Autodesk Fusion 360 part; units mm, degrees
(part 2 of 4)
  arc A532 (19.4796, 24.4743) -> (19.5304, 24.4743) centre (19.505, 24.4743) ccw
  arc A533 (21.1153, 25.5016) -> (20.7851, 25.1714) centre (21.1153, 25.1714) ccw
  arc A534 (22.3677, 26.8884) -> (22.4113, 26.9145) centre (22.3895, 26.9015) ccw
  arc A535 (22.0907, 25.1714) -> (22.0399, 25.1714) centre (22.0653, 25.1714) ccw
  arc A536 (23.3454, 24.2062) -> (23.3454, 24.1554) centre (23.3454, 24.1808) ccw
  arc A537 (19.7985, 24.94) -> (19.7985, 24.8892) centre (19.7985, 24.9146) ccw
  arc A538 (19.505, 24.4743) -> (19.7985, 24.1808) centre (19.7985, 24.4743) ccw
  arc A539 (20.2387, 24.1554) -> (20.2387, 24.2062) centre (20.2387, 24.1808) ccw
  arc A540 (21.5189, 24.1554) -> (21.5189, 24.2062) centre (21.5189, 24.1808) ccw
  arc A541 (20.7851, 24.2062) -> (20.7851, 24.1554) centre (20.7851, 24.1808) ccw
  line L151 (22.3895, 26.9014) -> (21.9492, 27.6352)
  arc A542 (19.4796, 24.6211) -> (19.5304, 24.6211) centre (19.505, 24.6211) ccw
  arc A543 (21.5189, 25.2081) -> (21.1153, 25.5016) centre (21.1153, 25.0774) ccw
  arc A544 (19.7985, 24.9146) -> (19.505, 24.6211) centre (19.7985, 24.6211) ccw
  arc A545 (21.0582, 26.3144) -> (21.3517, 26.6079) centre (21.0582, 26.6079) ccw
  line L152 (19.7985, 24.9146) -> (20.2387, 24.9146)
  arc A546 (20.2641, 25.5016) -> (20.2133, 25.5016) centre (20.2387, 25.5016) ccw
  arc A547 (22.1578, 24.8962) -> (22.1929, 24.933) centre (22.1754, 24.9146) ccw
  arc A548 (23.4748, 24.931) -> (23.4361, 24.8981) centre (23.4554, 24.9145) ccw
  arc A549 (22.3955, 25.527) -> (22.3955, 25.4762) centre (22.3955, 25.5016) ccw
  line L153 (20.2387, 24.1808) -> (19.7985, 24.1808)
  line L154 (20.2387, 24.9146) -> (20.2387, 25.5016)
  arc A550 (22.3955, 25.5016) -> (22.0653, 25.1714) centre (22.3955, 25.1714) ccw
  line L155 (22.1753, 24.9146) -> (22.799, 24.1808)
  arc A551 (23.7377, 27.6352) -> (23.6869, 27.6352) centre (23.7123, 27.6352) ccw
  line L156 (23.4555, 24.9146) -> (24.0792, 24.1808)
  arc A552 (23.438, 24.8962) -> (23.473, 24.933) centre (23.4555, 24.9146) ccw
  arc A553 (24.0598, 24.1643) -> (24.0986, 24.1973) centre (24.0792, 24.1808) ccw
  line L157 (20.7647, 26.3144) -> (21.0582, 26.3144)
  arc A554 (21.9238, 26.3144) -> (21.9746, 26.3144) centre (21.9492, 26.3144) ccw
  line L158 (24.0792, 27.6352) -> (23.3454, 27.6352)
  line L159 (21.3517, 26.6079) -> (21.3517, 27.3417)
  arc A555 (20.7597, 25.1714) -> (20.8105, 25.1714) centre (20.7851, 25.1714) ccw
  arc A556 (27.0866, 42.545) -> (27.1818, 42.1322) centre (28.0285, 42.5448) ccw
  arc A557 (27.1749, 42.8823) -> (27.1253, 42.8427) centre (27.1501, 42.8625) ccw
  arc A558 (26.0673, 42.9438) -> (26.0103, 42.9717) centre (26.0388, 42.9578) ccw
  arc A559 (20.2387, 24.8892) -> (20.2387, 24.94) centre (20.2387, 24.9146) ccw
  line L160 (27.6581, 42.2275) -> (27.1501, 42.8625)
  arc A560 (26.5786, 42.545) -> (26.4833, 42.9578) centre (25.6366, 42.5449) ccw
  arc A561 (25.4419, 42.7355) -> (25.3784, 42.7355) centre (25.4102, 42.7355) ccw
  arc A562 (22.799, 25.2081) -> (22.3955, 25.5016) centre (22.3955, 25.0775) ccw
  arc A563 (26.4548, 42.1462) -> (26.5118, 42.1183) centre (26.4833, 42.1322) ccw
  arc A564 (22.799, 24.1554) -> (22.799, 24.2062) centre (22.799, 24.1808) ccw
  arc A565 (20.2133, 24.9146) -> (20.2641, 24.9146) centre (20.2387, 24.9146) ccw
  line L161 (20.2387, 25.5016) -> (19.505, 25.5016)
  arc A566 (26.4533, 42.9475) -> (26.5133, 42.968) centre (26.4833, 42.9577) ccw
  arc A567 (27.1183, 42.545) -> (27.0548, 42.545) centre (27.0866, 42.545) ccw
  arc A568 (27.2103, 42.9438) -> (27.1533, 42.9717) centre (27.1818, 42.9578) ccw
  line L162 (28.5471, 43.1165) -> (28.5471, 41.9735)
  line L163 (28.8646, 42.8625) -> (28.5471, 43.1165)
  arc A569 (25.9118, 42.545) -> (25.9753, 42.545) centre (25.9436, 42.545) ccw
  arc A570 (27.4041, 42.0053) -> (27.4041, 41.9417) centre (27.4041, 41.9735) ccw
  arc A571 (19.7985, 24.2062) -> (19.7985, 24.1554) centre (19.7985, 24.1808) ccw
  arc A572 (26.6103, 42.545) -> (26.5468, 42.545) centre (26.5785, 42.545) ccw
  arc A573 (27.7533, 42.545) -> (27.6898, 42.545) centre (27.7216, 42.545) ccw
  arc A574 (28.5669, 43.1413) -> (28.5272, 43.0917) centre (28.547, 43.1165) ccw
  arc A575 (27.4041, 43.1165) -> (27.1818, 42.9578) centre (27.404, 42.8816) ccw
  arc A576 (27.6898, 42.545) -> (27.7533, 42.545) centre (27.7216, 42.545) ccw
  arc A577 (27.6263, 42.1322) -> (27.7216, 42.545) centre (26.7796, 42.5451) ccw
  arc A578 (27.4041, 43.1483) -> (27.4041, 43.0847) centre (27.4041, 43.1165) ccw
  arc A579 (28.8447, 42.8377) -> (28.8844, 42.8873) centre (28.8646, 42.8625) ccw
  arc A580 (26.2611, 43.1165) -> (26.0388, 42.9578) centre (26.261, 42.8816) ccw
  arc A581 (27.0548, 42.545) -> (27.1183, 42.545) centre (27.0866, 42.545) ccw
  arc A582 (27.5978, 42.1462) -> (27.6548, 42.1183) centre (27.6263, 42.1322) ccw
  arc A583 (24.9339, 42.545) -> (24.8704, 42.545) centre (24.9022, 42.545) ccw
  arc A584 (21.4947, 25.2003) -> (21.5431, 25.2159) centre (21.5189, 25.2081) ccw
  arc A585 (20.7851, 25.1714) -> (20.8952, 24.9146) centre (21.1397, 25.1714) ccw
  arc A586 (27.1818, 42.9578) -> (27.0866, 42.545) centre (28.0285, 42.5452) ccw
  arc A587 (27.1518, 42.968) -> (27.2118, 42.9475) centre (27.1818, 42.9577) ccw
  arc A588 (27.4041, 41.9417) -> (27.4041, 42.0053) centre (27.4041, 41.9735) ccw
  arc A589 (27.5963, 42.9475) -> (27.6563, 42.968) centre (27.6263, 42.9577) ccw
  arc A590 (28.2296, 42.0053) -> (28.2296, 41.9417) centre (28.2296, 41.9735) ccw
  arc A591 (26.0388, 42.9578) -> (25.9436, 42.545) centre (26.8855, 42.5452) ccw
  line L164 (19.505, 24.4743) -> (19.505, 24.6211)
  arc A592 (26.4833, 42.1322) -> (26.5786, 42.545) centre (25.6366, 42.5451) ccw
  arc A593 (27.6263, 42.9578) -> (27.4041, 43.1165) centre (27.4041, 42.8816) ccw
  arc A594 (26.2611, 43.0847) -> (26.2611, 43.1483) centre (26.2611, 43.1165) ccw
  line L165 (24.13, 43.1165) -> (24.0665, 43.1165)
  arc A595 (27.6563, 42.122) -> (27.5963, 42.1425) centre (27.6263, 42.1322) ccw
  arc A596 (27.2118, 42.1425) -> (27.1518, 42.122) centre (27.1818, 42.1322) ccw
  arc A597 (28.5153, 41.9735) -> (28.5788, 41.9735) centre (28.5471, 41.9735) ccw
  arc A598 (27.1818, 42.1322) -> (27.4041, 41.9735) centre (27.404, 42.2084) ccw
  arc A599 (27.7216, 42.545) -> (27.6263, 42.9578) centre (26.7796, 42.5449) ccw
  arc A600 (27.4041, 41.9735) -> (27.6263, 42.1322) centre (27.4041, 42.2084) ccw
  arc A601 (26.4833, 42.9578) -> (26.2611, 43.1165) centre (26.2611, 42.8816) ccw
  arc A602 (27.6333, 42.2077) -> (27.6829, 42.2473) centre (27.6581, 42.2275) ccw
  arc A603 (26.2611, 43.1483) -> (26.2611, 43.0847) centre (26.2611, 43.1165) ccw
  arc A604 (26.0088, 42.968) -> (26.0688, 42.9475) centre (26.0388, 42.9577) ccw
  arc A605 (26.5468, 42.545) -> (26.6103, 42.545) centre (26.5785, 42.545) ccw
  arc A606 (26.5118, 42.9717) -> (26.4548, 42.9438) centre (26.4833, 42.9578) ccw
  line L166 (20.8952, 24.9146) -> (21.5189, 24.1808)
  arc A607 (27.1533, 42.1183) -> (27.2103, 42.1462) centre (27.1818, 42.1322) ccw
  arc A608 (27.4041, 43.0847) -> (27.4041, 43.1483) centre (27.4041, 43.1165) ccw
  arc A609 (28.5788, 43.1165) -> (28.5153, 43.1165) centre (28.5471, 43.1165) ccw
  arc A610 (28.8646, 41.9417) -> (28.8646, 42.0053) centre (28.8646, 41.9735) ccw
  line L167 (28.8646, 41.9735) -> (28.2296, 41.9735)
  arc A611 (27.6548, 42.9717) -> (27.5978, 42.9438) centre (27.6263, 42.9578) ccw
  arc A612 (27.1699, 47.8403) -> (27.1302, 47.7907) centre (27.1501, 47.8155) ccw
  arc A613 (24.0665, 47.625) -> (23.876, 47.8155) centre (23.876, 47.625) ccw
  arc A614 (25.9753, 42.545) -> (25.9118, 42.545) centre (25.9436, 42.545) ccw
  line L168 (27.1501, 47.8155) -> (27.1501, 46.6725)
  line L169 (26.5151, 42.2275) -> (26.0071, 42.8625)
  arc A615 (24.8704, 41.9735) -> (24.9339, 41.9735) centre (24.9022, 41.9735) ccw
  arc A616 (25.1879, 47.4345) -> (25.1244, 47.4345) centre (25.1562, 47.4345) ccw
  arc A617 (26.2293, 46.8313) -> (26.3246, 47.244) centre (25.3829, 47.2441) ccw
  arc A618 (25.7213, 47.244) -> (25.6578, 47.244) centre (25.6896, 47.244) ccw
  arc A619 (23.876, 47.7837) -> (23.876, 47.8473) centre (23.876, 47.8155) ccw
  arc A620 (26.0071, 46.6407) -> (26.0071, 46.7043) centre (26.0071, 46.6725) ccw
  arc A621 (25.7563, 46.8173) -> (25.8133, 46.8452) centre (25.7848, 46.8313) ccw
  arc A622 (24.0983, 47.625) -> (24.0348, 47.625) centre (24.0666, 47.625) ccw
  arc A623 (25.0927, 42.7037) -> (25.0927, 42.7673) centre (25.0927, 42.7355) ccw
  arc A624 (24.0348, 47.625) -> (24.0983, 47.625) centre (24.0666, 47.625) ccw
  arc A625 (23.8125, 47.8473) -> (23.8125, 47.7837) centre (23.8125, 47.8155) ccw
  arc A626 (24.4475, 42.7037) -> (24.4475, 42.7673) centre (24.4475, 42.7355) ccw
  arc A627 (23.876, 47.8473) -> (23.876, 47.7837) centre (23.876, 47.8155) ccw
  line L170 (27.4676, 47.5615) -> (27.1501, 47.8155)
  arc A628 (24.13, 43.0847) -> (24.13, 43.1483) centre (24.13, 43.1165) ccw
  line L171 (25.4102, 42.7355) -> (25.0927, 42.7355)
  line L172 (24.3205, 41.9735) -> (24.3205, 42.926)
  arc A629 (25.3784, 41.9735) -> (25.4419, 41.9735) centre (25.4102, 41.9735) ccw
  arc A630 (24.3523, 42.926) -> (24.2888, 42.926) centre (24.3206, 42.926) ccw
  arc A631 (26.4903, 42.2077) -> (26.5399, 42.2473) centre (26.5151, 42.2275) ccw
  line L173 (24.9022, 42.545) -> (24.9022, 41.9735)
  line L174 (24.4475, 42.7355) -> (24.0665, 42.7355)
  arc A632 (24.0665, 42.7673) -> (24.0665, 42.7037) centre (24.0665, 42.7355) ccw
  arc A633 (26.0388, 42.1322) -> (26.2611, 41.9735) centre (26.261, 42.2084) ccw
  line L175 (25.4102, 41.9735) -> (25.4102, 42.7355)
  arc A634 (24.8704, 42.545) -> (24.9339, 42.545) centre (24.9022, 42.545) ccw
  arc A635 (26.2611, 41.9735) -> (26.4833, 42.1322) centre (26.2611, 42.2084) ccw
  arc A636 (25.0927, 42.7673) -> (25.0927, 42.7037) centre (25.0927, 42.7355) ccw
  arc A637 (25.7779, 47.5813) -> (25.7283, 47.5417) centre (25.7531, 47.5615) ccw
  arc A638 (24.6482, 46.7043) -> (24.6482, 46.6407) centre (24.6482, 46.6725) ccw
  arc A639 (25.6896, 47.244) -> (25.7848, 46.8313) centre (26.6313, 47.2439) ccw
  arc A640 (25.8133, 47.6428) -> (25.7563, 47.6707) centre (25.7848, 47.6567) ccw
  arc A641 (24.2888, 41.9735) -> (24.3523, 41.9735) centre (24.3206, 41.9735) ccw
  arc A642 (24.3205, 42.926) -> (24.13, 43.1165) centre (24.13, 42.926) ccw
  arc A643 (24.2888, 42.926) -> (24.3523, 42.926) centre (24.3206, 42.926) ccw
  arc A644 (24.13, 43.1483) -> (24.13, 43.0847) centre (24.13, 43.1165) ccw
  line L176 (27.4676, 46.6725) -> (26.8326, 46.6725)
  arc A645 (25.7848, 47.6568) -> (25.6896, 47.244) centre (26.6315, 47.2442) ccw
  arc A646 (26.3246, 47.244) -> (26.2293, 47.6568) centre (25.3826, 47.2439) ccw
  arc A647 (27.1183, 46.6725) -> (27.1818, 46.6725) centre (27.1501, 46.6725) ccw
  arc A648 (25.6578, 47.244) -> (25.7213, 47.244) centre (25.6896, 47.244) ccw
  arc A649 (26.2008, 46.8452) -> (26.2578, 46.8173) centre (26.2293, 46.8313) ccw
  line L177 (24.0665, 46.6725) -> (24.0665, 47.625)
  arc A650 (27.1818, 47.8155) -> (27.1183, 47.8155) centre (27.1501, 47.8155) ccw
  arc A651 (24.0348, 46.6725) -> (24.0983, 46.6725) centre (24.0666, 46.6725) ccw
  arc A652 (26.0103, 42.1183) -> (26.0673, 42.1462) centre (26.0388, 42.1322) ccw
  line L178 (24.9657, 46.6725) -> (24.6482, 46.6725)
  arc A653 (24.6164, 46.6725) -> (24.6799, 46.6725) centre (24.6482, 46.6725) ccw
  arc A654 (25.7548, 47.667) -> (25.8148, 47.6465) centre (25.7848, 47.6568) ccw
  arc A655 (27.4477, 47.5367) -> (27.4874, 47.5863) centre (27.4675, 47.5615) ccw
  arc A656 (25.9436, 42.545) -> (26.0388, 42.1322) centre (26.8855, 42.5448) ccw
  arc A657 (25.0927, 42.7355) -> (24.9022, 42.545) centre (25.0927, 42.545) ccw
  arc A658 (25.4102, 42.7037) -> (25.4102, 42.7673) centre (25.4102, 42.7355) ccw
  arc A659 (26.0688, 42.1425) -> (26.0088, 42.122) centre (26.0388, 42.1322) ccw
  arc A660 (26.2611, 42.0053) -> (26.2611, 41.9417) centre (26.2611, 41.9735) ccw
  arc A661 (26.2611, 41.9417) -> (26.2611, 42.0053) centre (26.2611, 41.9735) ccw
  arc A662 (26.5133, 42.122) -> (26.4533, 42.1425) centre (26.4833, 42.1322) ccw
  arc A663 (26.0319, 42.8823) -> (25.9823, 42.8427) centre (26.0071, 42.8625) ccw
  arc A664 (24.0665, 43.1483) -> (24.0665, 43.0847) centre (24.0665, 43.1165) ccw
  arc A665 (9.6838, 38.608) -> (9.7472, 38.608) centre (9.7155, 38.608) ccw
  arc A666 (10.2252, 39.0105) -> (10.2853, 39.031) centre (10.2553, 39.0207) ccw
  arc A667 (26.0071, 47.7837) -> (26.0071, 47.8473) centre (26.0071, 47.8155) ccw
  arc A668 (11.3983, 39.0207) -> (11.176, 39.1795) centre (11.176, 38.9445) ccw
  arc A669 (24.9657, 46.6725) -> (25.1562, 46.863) centre (24.9657, 46.863) ccw
  line L179 (26.2611, 46.9265) -> (25.7531, 47.5615)
  arc A670 (10.033, 38.0365) -> (10.2553, 38.1953) centre (10.033, 38.2715) ccw
  arc A671 (10.2853, 38.185) -> (10.2252, 38.2055) centre (10.2553, 38.1953) ccw
  arc A672 (11.4618, 38.608) -> (11.5252, 38.608) centre (11.4935, 38.608) ccw
  arc A673 (11.3983, 38.1953) -> (11.4935, 38.608) centre (10.5518, 38.6079) ccw
  arc A674 (11.176, 38.0683) -> (11.176, 38.0048) centre (11.176, 38.0366) ccw
  arc A675 (9.8393, 39.0068) -> (9.7822, 39.0347) centre (9.8107, 39.0207) ccw
  arc A676 (12.3388, 39.2043) -> (12.2992, 39.1547) centre (12.319, 39.1795) ccw
  line L180 (12.6365, 38.9255) -> (12.319, 39.1795)
  arc A677 (11.5252, 38.608) -> (11.4618, 38.608) centre (11.4935, 38.608) ccw
  arc A678 (11.176, 39.2113) -> (11.176, 39.1478) centre (11.176, 39.1795) ccw
  arc A679 (11.4935, 38.608) -> (11.3983, 39.0207) centre (10.5518, 38.6081) ccw
  arc A680 (12.6365, 38.0048) -> (12.6365, 38.0683) centre (12.6365, 38.0366) ccw
  arc A681 (26.0071, 46.7043) -> (26.0071, 46.6407) centre (26.0071, 46.6725) ccw
  line L181 (23.876, 47.8155) -> (23.8125, 47.8155)
  arc A682 (26.0071, 47.8473) -> (26.0071, 47.7837) centre (26.0071, 47.8155) ccw
  arc A683 (10.2553, 39.0207) -> (10.033, 39.1795) centre (10.033, 38.9445) ccw
  arc A684 (26.2578, 47.6707) -> (26.2008, 47.6428) centre (26.2293, 47.6568) ccw
  arc A685 (10.3822, 38.608) -> (10.3188, 38.608) centre (10.3505, 38.608) ccw
  arc A686 (10.9252, 38.1813) -> (10.9823, 38.2092) centre (10.9538, 38.1953) ccw
  arc A687 (25.1879, 46.863) -> (25.1244, 46.863) centre (25.1562, 46.863) ccw
  arc A688 (11.176, 39.1795) -> (10.9538, 39.0207) centre (11.176, 38.9446) ccw
  arc A689 (10.2267, 38.2092) -> (10.2838, 38.1813) centre (10.2553, 38.1953) ccw
  arc A690 (26.2363, 46.9067) -> (26.2859, 46.9463) centre (26.2611, 46.9265) ccw
  arc A691 (11.176, 39.1478) -> (11.176, 39.2113) centre (11.176, 39.1795) ccw
  arc A692 (10.9838, 38.2055) -> (10.9237, 38.185) centre (10.9537, 38.1953) ccw
  arc A693 (26.0071, 47.8155) -> (25.7848, 47.6568) centre (26.007, 47.5806) ccw
  line L182 (24.1935, 47.4345) -> (23.8125, 47.4345)
  arc A694 (10.8585, 38.608) -> (10.9538, 38.1953) centre (11.8002, 38.6081) ccw
  arc A695 (11.3697, 38.2092) -> (11.4268, 38.1813) centre (11.3983, 38.1953) ccw
  arc A696 (11.176, 38.0048) -> (11.176, 38.0683) centre (11.176, 38.0366) ccw
  arc A697 (11.4268, 39.0347) -> (11.3697, 39.0068) centre (11.3983, 39.0207) ccw
  arc A698 (25.7848, 46.8313) -> (26.0071, 46.6725) centre (26.0071, 46.9075) ccw
  arc A699 (26.2593, 46.821) -> (26.1993, 46.8415) centre (26.2293, 46.8313) ccw
  arc A700 (26.2928, 47.244) -> (26.3563, 47.244) centre (26.3246, 47.244) ccw
  arc A701 (26.2293, 47.6568) -> (26.0071, 47.8155) centre (26.0071, 47.5806) ccw
  arc A702 (26.0071, 46.6725) -> (26.2293, 46.8313) centre (26.0071, 46.9074) ccw
  arc A703 (10.2553, 38.1953) -> (10.3505, 38.608) centre (9.4088, 38.6079) ccw
  arc A704 (11.3682, 39.0105) -> (11.4283, 39.031) centre (11.3983, 39.0207) ccw
  arc A705 (24.1935, 47.4027) -> (24.1935, 47.4663) centre (24.1935, 47.4345) ccw
  arc A706 (12.2873, 38.0365) -> (12.3508, 38.0365) centre (12.3191, 38.0365) ccw
  arc A707 (10.8268, 38.608) -> (10.8902, 38.608) centre (10.8585, 38.608) ccw
  arc A708 (10.9823, 39.0068) -> (10.9252, 39.0347) centre (10.9537, 39.0207) ccw
  arc A709 (26.1993, 47.6465) -> (26.2593, 47.667) centre (26.2293, 47.6568) ccw
  arc A710 (10.033, 38.0683) -> (10.033, 38.0048) centre (10.033, 38.0366) ccw
  arc A711 (25.8148, 46.8415) -> (25.7548, 46.821) centre (25.7848, 46.8313) ccw
  arc A712 (11.4283, 38.185) -> (11.3682, 38.2055) centre (11.3983, 38.1953) ccw
  arc A713 (10.2838, 39.0347) -> (10.2267, 39.0068) centre (10.2553, 39.0207) ccw
  arc A714 (10.9538, 39.0207) -> (10.8585, 38.608) centre (11.8002, 38.6079) ccw
  arc A715 (24.6799, 47.4345) -> (24.6164, 47.4345) centre (24.6482, 47.4345) ccw
  arc A716 (23.8125, 47.4663) -> (23.8125, 47.4027) centre (23.8125, 47.4345) ccw
  arc A717 (24.9657, 46.7043) -> (24.9657, 46.6407) centre (24.9657, 46.6725) ccw
  line L183 (24.6482, 46.6725) -> (24.6482, 47.4345)
  arc A718 (25.1244, 46.863) -> (25.1879, 46.863) centre (25.1562, 46.863) ccw
  arc A719 (24.9657, 46.6407) -> (24.9657, 46.7043) centre (24.9657, 46.6725) ccw
  arc A720 (27.4676, 46.6407) -> (27.4676, 46.7043) centre (27.4676, 46.6725) ccw
  arc A721 (26.8326, 46.7043) -> (26.8326, 46.6407) centre (26.8326, 46.6725) ccw
  arc A722 (26.3563, 47.244) -> (26.2928, 47.244) centre (26.3246, 47.244) ccw
  line L184 (25.1562, 47.4345) -> (25.1562, 46.863)
  arc A723 (8.2194, 38.7668) -> (8.2194, 38.8303) centre (8.2194, 38.7986) ccw
  line L185 (8.9916, 38.0365) -> (8.6741, 38.0365)
  arc A724 (9.8038, 38.9453) -> (9.7542, 38.9057) centre (9.779, 38.9255) ccw
  line L186 (12.319, 39.1795) -> (12.319, 38.0365)
  arc A725 (8.0607, 38.989) -> (8.1242, 38.989) centre (8.0925, 38.989) ccw
  arc A726 (10.3188, 38.608) -> (10.3822, 38.608) centre (10.3505, 38.608) ccw
  arc A727 (12.6167, 38.9007) -> (12.6563, 38.9503) centre (12.6365, 38.9255) ccw
  arc A728 (8.0607, 38.0365) -> (8.1242, 38.0365) centre (8.0925, 38.0365) ccw
  arc A729 (10.2622, 38.2707) -> (10.3118, 38.3103) centre (10.287, 38.2905) ccw
  arc A730 (9.1503, 38.227) -> (9.2139, 38.227) centre (9.1821, 38.227) ccw
  line L187 (8.0924, 38.0365) -> (8.0924, 38.989)
  arc A731 (10.033, 39.1795) -> (9.8108, 39.0207) centre (10.033, 38.9446) ccw
  arc A732 (8.6424, 38.0365) -> (8.7059, 38.0365) centre (8.6742, 38.0365) ccw
  arc A733 (8.9916, 38.0683) -> (8.9916, 38.0048) centre (8.9916, 38.0366) ccw
  arc A734 (9.8408, 38.2055) -> (9.7807, 38.185) centre (9.8107, 38.1953) ccw
  line L188 (12.6365, 38.0365) -> (12.0015, 38.0365)
  arc A735 (9.7822, 38.1813) -> (9.8393, 38.2092) centre (9.8107, 38.1953) ccw
  arc A736 (8.6741, 38.0683) -> (8.6741, 38.0048) centre (8.6741, 38.0366) ccw
  arc A737 (8.9916, 38.0048) -> (8.9916, 38.0683) centre (8.9916, 38.0366) ccw
  arc A738 (7.8384, 39.2113) -> (7.8384, 39.1478) centre (7.8384, 39.1795) ccw
  line L189 (21.8689, 40.0242) -> (22.9191, 40.5364)
  arc A739 (10.9538, 38.1953) -> (11.176, 38.0365) centre (11.176, 38.2714) ccw
  arc A740 (9.7807, 39.031) -> (9.8408, 39.0105) centre (9.8107, 39.0207) ccw
  arc A741 (9.2139, 38.7985) -> (9.1503, 38.7985) centre (9.1821, 38.7985) ccw
  arc A742 (10.8902, 38.608) -> (10.8268, 38.608) centre (10.8585, 38.608) ccw
  arc A743 (8.1242, 38.989) -> (8.0607, 38.989) centre (8.0925, 38.989) ccw
  arc A744 (7.8384, 38.8303) -> (7.8384, 38.7668) centre (7.8384, 38.7986) ccw
  line L190 (7.9019, 39.1795) -> (7.8384, 39.1795)
  line L191 (11.43, 38.2905) -> (10.922, 38.9255)
  arc A745 (21.7517, 41.2431) -> (21.7974, 41.2654) centre (21.7746, 41.2543) ccw
  arc A746 (22.3128, 40.2407) -> (22.3585, 40.263) centre (22.3357, 40.2518) ccw
  arc A747 (20.6441, 42.5199) -> (20.6778, 42.4819) centre (20.661, 42.5009) ccw
  arc A748 (12.0015, 38.0683) -> (12.0015, 38.0048) centre (12.0015, 38.0366) ccw
  arc A749 (20.5828, 43.4016) -> (20.605, 43.3559) centre (20.5939, 43.3788) ccw
  arc A750 (8.7059, 38.7985) -> (8.6424, 38.7985) centre (8.6742, 38.7985) ccw
  arc A751 (9.8108, 39.0207) -> (9.7155, 38.608) centre (10.6572, 38.6079) ccw
  arc A752 (19.3441, 45.143) -> (19.3897, 45.1653) centre (19.3669, 45.1542) ccw
  arc A753 (22.7996, 40.8392) -> (22.754, 40.817) centre (22.7768, 40.8281) ccw
  arc A754 (21.1016, 43.6704) -> (21.0794, 43.716) centre (21.0905, 43.6932) ccw
  arc A755 (22.754, 40.817) -> (22.7996, 40.8392) centre (22.7768, 40.8281) ccw
  arc A756 (22.7768, 40.8281) -> (22.1934, 40.5435) centre (22.4851, 40.6858) ccw
  arc A757 (10.9237, 39.031) -> (10.9838, 39.0105) centre (10.9537, 39.0207) ccw
  line L192 (8.2194, 38.7985) -> (7.8384, 38.7985)
  arc A758 (7.9019, 39.2113) -> (7.9019, 39.1478) centre (7.9019, 39.1795) ccw
  arc A759 (22.1706, 40.5324) -> (22.2162, 40.5547) centre (22.1934, 40.5436) ccw
  arc A760 (22.8962, 40.5252) -> (22.9419, 40.5475) centre (22.919, 40.5364) ccw
  arc A761 (8.0924, 38.989) -> (7.9019, 39.1795) centre (7.9019, 38.989) ccw
  arc A762 (10.033, 38.0048) -> (10.033, 38.0683) centre (10.033, 38.0366) ccw
  arc A763 (9.2139, 38.227) -> (9.1503, 38.227) centre (9.1821, 38.227) ccw
  arc A764 (10.033, 39.1478) -> (10.033, 39.2113) centre (10.033, 39.1795) ccw
  arc A765 (11.4052, 38.2707) -> (11.4548, 38.3103) centre (11.43, 38.2905) ccw
  arc A766 (9.8108, 38.1953) -> (10.033, 38.0365) centre (10.033, 38.2714) ccw
  arc A767 (8.9916, 38.0365) -> (9.1821, 38.227) centre (8.9916, 38.227) ccw
  line L193 (8.6741, 38.0365) -> (8.6741, 38.7985)
  line L194 (9.1821, 38.7985) -> (9.1821, 38.227)
  arc A768 (10.3505, 38.608) -> (10.2553, 39.0207) centre (9.4088, 38.6081) ccw
  arc A769 (12.3508, 39.1795) -> (12.2873, 39.1795) centre (12.3191, 39.1795) ccw
  arc A770 (11.176, 38.0365) -> (11.3983, 38.1953) centre (11.176, 38.2715) ccw
  arc A771 (10.9468, 38.9453) -> (10.8972, 38.9057) centre (10.922, 38.9255) ccw
  arc A772 (10.033, 39.2113) -> (10.033, 39.1478) centre (10.033, 39.1795) ccw
  arc A773 (9.7155, 38.608) -> (9.8108, 38.1953) centre (10.6572, 38.6081) ccw
  arc A774 (9.7472, 38.608) -> (9.6838, 38.608) centre (9.7155, 38.608) ccw
  arc A775 (7.9019, 39.1478) -> (7.9019, 39.2113) centre (7.9019, 39.1795) ccw
  line L195 (10.287, 38.2905) -> (9.779, 38.9255)
  line L196 (21.5688, 43.3048) -> (20.661, 42.5009)
  arc A776 (21.7256, 42.6873) -> (21.7478, 42.6416) centre (21.7367, 42.6645) ccw
  arc A777 (20.874, 44.1371) -> (20.8517, 44.1828) centre (20.8629, 44.16) ccw
  line L197 (22.1934, 40.5435) -> (22.3357, 40.2518)
  arc A778 (22.1647, 40.5765) -> (22.1652, 40.6273) centre (22.165, 40.6019) ccw
  line L198 (22.9191, 40.5364) -> (22.7768, 40.8281)
  arc A779 (21.0794, 43.716) -> (21.1016, 43.6704) centre (21.0905, 43.6932) ccw
  arc A780 (18.5003, 46.873) -> (18.546, 46.8952) centre (18.5232, 46.8841) ccw
  arc A781 (18.8825, 46.2053) -> (18.8368, 46.183) centre (18.8597, 46.1942) ccw
  line L199 (19.3157, 45.8514) -> (19.4324, 45.9083)
  line L200 (18.9464, 46.1643) -> (18.918, 46.2226)
  arc A782 (19.527, 47.121) -> (19.5733, 47.3963) centre (19.3575, 47.2911) ccw
  arc A783 (19.3278, 47.5294) -> (18.9059, 47.4319) centre (19.3281, 46.5666) ccw
  arc A784 (21.8578, 40.047) -> (21.8801, 40.0014) centre (21.8689, 40.0242) ccw
  arc A785 (19.7723, 44.3229) -> (19.7946, 44.2773) centre (19.7834, 44.3001) ccw
  arc A786 (22.9302, 40.5136) -> (22.9079, 40.5592) centre (22.919, 40.5364) ccw
  arc A787 (19.2016, 46.8257) -> (19.1794, 46.8713) centre (19.1905, 46.8485) ccw
  arc A788 (20.3205, 43.9394) -> (20.2982, 43.985) centre (20.3093, 43.9622) ccw
  arc A789 (19.7606, 44.289) -> (19.8063, 44.3112) centre (19.7835, 44.3001) ccw
  arc A790 (21.0905, 43.6932) -> (20.8629, 44.1599) centre (20.9767, 43.9265) ccw
  line L201 (20.3669, 44.5846) -> (20.1961, 44.9347)
  arc A791 (20.3093, 43.9622) -> (20.5939, 43.3788) centre (20.4516, 43.6705) ccw
  arc A792 (20.219, 44.9458) -> (20.1733, 44.9236) centre (20.1961, 44.9347) ccw
  arc A793 (18.4815, 49.5768) -> (18.5272, 49.599) centre (18.5043, 49.5879) ccw
  arc A794 (18.1216, 49.0401) -> (18.4581, 49.3126) centre (17.6995, 49.9054) ccw
  line L202 (18.5678, 47.829) -> (18.2263, 48.5291)
  arc A795 (19.3157, 45.8514) -> (19.1962, 45.5042) centre (19.4296, 45.618) ccw
  arc A796 (18.546, 46.8952) -> (18.5003, 46.873) centre (18.5232, 46.8841) ccw
  arc A797 (18.5694, 47.1594) -> (18.5231, 46.8841) centre (18.739, 46.9893) ccw
  arc A798 (19.5505, 47.3852) -> (19.5961, 47.4074) centre (19.5733, 47.3963) ccw
  line L203 (21.7745, 41.2542) -> (21.4331, 41.9543)
  line L204 (20.8336, 44.8123) -> (20.6059, 45.279)
  arc A799 (18.2492, 48.5403) -> (18.2035, 48.518) centre (18.2263, 48.5292) ccw
  arc A800 (20.605, 43.3559) -> (20.5828, 43.4016) centre (20.5939, 43.3788) ccw
  line L205 (19.5558, 44.7668) -> (19.7834, 44.3001)
  arc A801 (21.8306, 42.7102) -> (21.8762, 42.7325) centre (21.8534, 42.7214) ccw
  arc A802 (19.7796, 45.7888) -> (19.4324, 45.9083) centre (19.5462, 45.6749) ccw
  arc A803 (19.5786, 44.778) -> (19.533, 44.7557) centre (19.5558, 44.7668) ccw
  arc A804 (21.5846, 40.633) -> (21.5841, 40.5822) centre (21.5843, 40.6076) ccw
  arc A805 (19.3268, 45.8286) -> (19.3046, 45.8742) centre (19.3157, 45.8514) ccw
  arc A806 (19.3046, 45.8742) -> (19.3268, 45.8286) centre (19.3157, 45.8514) ccw
  line L206 (19.3669, 45.1542) -> (19.1962, 45.5042)
  arc A807 (21.5917, 43.3159) -> (21.546, 43.2937) centre (21.5688, 43.3048) ccw
  line L207 (21.7367, 42.6645) -> (21.8534, 42.7214)
  arc A808 (21.8645, 42.6985) -> (21.8423, 42.7442) centre (21.8534, 42.7214) ccw
  arc A809 (19.4435, 45.8855) -> (19.4212, 45.9311) centre (19.4323, 45.9083) ccw
  arc A810 (20.6288, 45.2901) -> (20.5831, 45.2679) centre (20.6059, 45.279) ccw
  arc A811 (18.5494, 47.1751) -> (18.5894, 47.1438) centre (18.5694, 47.1594) ccw
  arc A812 (20.8517, 44.1828) -> (20.874, 44.1371) centre (20.8629, 44.16) ccw
  arc A813 (21.5857, 43.2858) -> (21.552, 43.3238) centre (21.5688, 43.3048) ccw
  arc A814 (20.2982, 43.985) -> (20.3205, 43.9394) centre (20.3093, 43.9622) ccw
  arc A815 (19.219, 45.5153) -> (19.1733, 45.4931) centre (19.1962, 45.5042) ccw
  arc A816 (20.5939, 43.3788) -> (20.3093, 43.9622) centre (20.4516, 43.6705) ccw
  arc A817 (19.7567, 45.7776) -> (19.8024, 45.7999) centre (19.7796, 45.7888) ccw
  arc A818 (21.4559, 41.9655) -> (21.4103, 41.9432) centre (21.4331, 41.9543) ccw
  arc A819 (20.8108, 44.8011) -> (20.8564, 44.8234) centre (20.8336, 44.8123) ccw
  line L208 (21.5844, 40.6076) -> (22.1649, 40.6019)
  line L209 (19.7834, 44.3001) -> (20.8336, 44.8123)
  arc A820 (20.8629, 44.1599) -> (21.0905, 43.6932) centre (20.9767, 43.9265) ccw
  arc A821 (20.8447, 44.7894) -> (20.8225, 44.8351) centre (20.8336, 44.8123) ccw
  line L210 (21.8534, 42.7214) -> (21.5688, 43.3048)
  arc A822 (22.2162, 40.5547) -> (22.1706, 40.5324) centre (22.1934, 40.5436) ccw
  arc A823 (20.344, 44.5735) -> (20.3897, 44.5958) centre (20.3669, 44.5847) ccw
  arc A824 (19.1733, 45.4931) -> (19.219, 45.5153) centre (19.1962, 45.5042) ccw
  arc A825 (18.9291, 46.1998) -> (18.9069, 46.2454) centre (18.918, 46.2226) ccw
  arc A826 (19.3278, 47.504) -> (19.3278, 47.5547) centre (19.3278, 47.5294) ccw
  arc A827 (18.2558, 49.7462) -> (18.2621, 49.6958) centre (18.259, 49.721) ccw
  line L211 (18.8596, 46.1942) -> (18.8881, 46.1358)
  arc A828 (19.5961, 47.4074) -> (19.5505, 47.3852) centre (19.5733, 47.3963) ccw
  arc A829 (17.1587, 49.8296) -> (17.1365, 49.8753) centre (17.1476, 49.8525) ccw
  arc A830 (18.9171, 47.4091) -> (18.8948, 47.4547) centre (18.906, 47.4319) ccw
  line L212 (18.8881, 46.1358) -> (18.9464, 46.1643)
  arc A831 (17.4542, 49.0757) -> (17.6997, 48.9427) centre (17.6701, 49.1811) ccw
  arc A832 (18.9059, 47.4319) -> (18.5694, 47.1594) centre (19.328, 46.5666) ccw
  arc A833 (20.3942, 45.6552) -> (20.4399, 45.6775) centre (20.4171, 45.6664) ccw
  line L213 (18.918, 46.2226) -> (18.8596, 46.1942)
  arc A834 (18.7686, 46.7764) -> (18.7686, 46.7256) centre (18.7686, 46.751) ccw
  arc A835 (18.1801, 49.6966) -> (18.1342, 49.7183) centre (18.1572, 49.7075) ccw
  arc A836 (17.3305, 50.868) -> (17.2849, 50.8457) centre (17.3077, 50.8568) ccw
  arc A837 (17.6997, 48.9427) -> (18.1216, 49.0401) centre (17.6996, 49.9054) ccw
  arc A838 (19.5733, 47.3963) -> (19.3278, 47.5294) centre (19.3574, 47.291) ccw
  arc A839 (19.1905, 46.8485) -> (19.527, 47.121) centre (18.7684, 47.7138) ccw
  arc A840 (19.8024, 45.7999) -> (19.7567, 45.7776) centre (19.7796, 45.7888) ccw
  line L214 (20.417, 45.6663) -> (20.1325, 46.2498)
  arc A841 (17.8482, 49.6007) -> (17.8259, 49.6463) centre (17.8371, 49.6235) ccw
  arc A842 (17.1872, 49.7713) -> (17.1649, 49.8169) centre (17.176, 49.7941) ccw
  arc A843 (18.2589, 49.721) -> (17.837, 49.6235) centre (18.2592, 48.7582) ccw
  arc A844 (18.9576, 46.1414) -> (18.9353, 46.1871) centre (18.9464, 46.1642) ccw
  line L215 (19.9503, 45.4387) -> (20.417, 45.6663)
  arc A845 (18.1104, 49.0629) -> (18.1327, 49.0173) centre (18.1215, 49.0401) ccw
  arc A846 (19.547, 47.1053) -> (19.507, 47.1366) centre (19.527, 47.1209) ccw
  arc A847 (19.3247, 47.5546) -> (19.331, 47.5041) centre (19.3279, 47.5294) ccw
  arc A848 (18.5873, 47.1415) -> (18.5515, 47.1774) centre (18.5694, 47.1594) ccw
  arc A849 (18.2589, 49.6956) -> (18.2589, 49.7464) centre (18.2589, 49.721) ccw
  arc A850 (18.5231, 46.8841) -> (18.7686, 46.751) centre (18.739, 46.9894) ccw
  arc A851 (18.9408, 46.2337) -> (18.8952, 46.2115) centre (18.918, 46.2226) ccw
  arc A852 (17.8259, 49.6463) -> (17.8482, 49.6007) centre (17.8371, 49.6235) ccw
  arc A853 (18.877, 46.1586) -> (18.8992, 46.113) centre (18.8881, 46.1358) ccw
  arc A854 (19.2491, 47.505) -> (19.2031, 47.5267) centre (19.2261, 47.5159) ccw
  arc A855 (19.5091, 47.1389) -> (19.545, 47.103) centre (19.527, 47.1209) ccw
  line L216 (18.8703, 46.7646) -> (19.2261, 47.5158)
  arc A856 (20.1553, 46.2609) -> (20.1097, 46.2386) centre (20.1325, 46.2497) ccw
  arc A857 (18.8948, 47.4547) -> (18.9171, 47.4091) centre (18.906, 47.4319) ccw
  arc A858 (18.8474, 46.7754) -> (18.8933, 46.7537) centre (18.8704, 46.7645) ccw
  arc A859 (18.4402, 49.3306) -> (18.476, 49.2946) centre (18.4581, 49.3126) ccw
  arc A860 (19.9275, 45.4276) -> (19.9731, 45.4498) centre (19.9503, 45.4387) ccw
  arc A861 (20.4282, 45.6435) -> (20.4059, 45.6892) centre (20.417, 45.6664) ccw
  arc A862 (18.4581, 49.3126) -> (18.5044, 49.5879) centre (18.2886, 49.4827) ccw
  arc A863 (18.5044, 49.5879) -> (18.2589, 49.721) centre (18.2885, 49.4826) ccw
  arc A864 (19.4213, 45.9311) -> (19.4435, 45.8855) centre (19.4324, 45.9083) ccw
  arc A865 (18.7686, 46.751) -> (19.1905, 46.8485) centre (18.7683, 47.7138) ccw
  line L217 (19.7796, 45.7888) -> (19.9503, 45.4387)
  arc A866 (18.8485, 46.217) -> (18.8708, 46.1713) centre (18.8596, 46.1942) ccw
  arc A867 (18.545, 47.8179) -> (18.5906, 47.8402) centre (18.5678, 47.8291) ccw
  arc A868 (17.1066, 49.7885) -> (17.1288, 49.7428) centre (17.1177, 49.7657) ccw
  arc A869 (16.9717, 50.9536) -> (16.9494, 50.9992) centre (16.9605, 50.9764) ccw
  arc A870 (17.7785, 48.967) -> (17.8244, 48.9453) centre (17.8015, 48.9562) ccw
  arc A871 (16.8722, 50.2111) -> (16.9179, 50.2334) centre (16.8951, 50.2223) ccw
  arc A872 (17.0949, 49.7545) -> (17.1405, 49.7768) centre (17.1177, 49.7657) ccw
  arc A873 (18.7717, 46.7258) -> (18.7655, 46.7762) centre (18.7686, 46.751) ccw
  arc A874 (19.9392, 45.4615) -> (19.9614, 45.4159) centre (19.9503, 45.4387) ccw
  arc A875 (18.9236, 46.1531) -> (18.9693, 46.1754) centre (18.9465, 46.1643) ccw
  arc A876 (19.1794, 46.8713) -> (19.2016, 46.8257) centre (19.1905, 46.8485) ccw
  arc A877 (18.4781, 49.2969) -> (18.4381, 49.3282) centre (18.4581, 49.3125) ccw
  arc A878 (18.8653, 46.1247) -> (18.9109, 46.1469) centre (18.8881, 46.1358) ccw
  line L218 (17.3077, 50.8568) -> (17.4784, 50.5068)
  arc A879 (18.5272, 49.599) -> (18.4815, 49.5768) centre (18.5044, 49.5879) ccw
  arc A880 (17.5184, 49.3331) -> (17.4825, 49.369) centre (17.5004, 49.3511) ccw
  arc A881 (18.1327, 49.0173) -> (18.1104, 49.0629) centre (18.1216, 49.0401) ccw
  arc A882 (24.607, 10.9753) -> (24.5674, 11.007) centre (24.5872, 10.9912) ccw
  line L219 (17.1476, 49.8525) -> (17.0893, 49.824)
  line L220 (17.8014, 48.9562) -> (18.1572, 49.7074)
  line L221 (24.5872, 10.9911) -> (23.6982, 10.9911)
  arc A883 (24.3112, 12.0473) -> (24.2705, 12.0778) centre (24.2908, 12.0626) ccw
  line L222 (23.6982, 12.0626) -> (24.118, 11.8403)
  arc A884 (17.6997, 48.968) -> (17.6997, 48.9173) centre (17.6997, 48.9427) ccw
  arc A885 (23.6728, 10.7442) -> (23.7236, 10.7442) centre (23.6982, 10.7442) ccw
  arc A886 (1.2573, 32.5538) -> (1.1811, 32.5538) centre (1.2192, 32.5538) ccw
  arc A887 (17.4673, 50.5296) -> (17.4896, 50.484) centre (17.4785, 50.5068) ccw
  arc A888 (16.9494, 50.9992) -> (16.9717, 50.9536) centre (16.9605, 50.9764) ccw
  line L223 (1.2192, 33.4462) -> (2.3029, 33.4462)
  arc A889 (17.4556, 50.4957) -> (17.5013, 50.5179) centre (17.4785, 50.5068) ccw
  line L224 (23.6982, 10.7442) -> (23.6982, 11.2381)
  arc A890 (2.3029, 32.0642) -> (2.3029, 32.1404) centre (2.3029, 32.1023) ccw
  arc A891 (17.9563, 50.7116) -> (17.934, 50.7573) centre (17.9451, 50.7344) ccw
  arc A892 (17.7028, 48.9174) -> (17.6965, 48.9679) centre (17.6997, 48.9427) ccw
  arc A893 (23.7236, 11.2381) -> (23.6728, 11.2381) centre (23.6982, 11.2381) ccw
  arc A894 (17.3077, 50.8568) -> (16.9605, 50.9764) centre (17.0743, 50.743) ccw
  arc A895 (17.4805, 49.3667) -> (17.5205, 49.3354) centre (17.5005, 49.3511) ccw
  line L225 (24.3896, 10.7442) -> (24.5872, 10.9911)
  line L226 (23.6982, 11.6675) -> (24.5872, 11.6675)
  arc A896 (16.7015, 50.5612) -> (16.7471, 50.5834) centre (16.7243, 50.5723) ccw
  arc A897 (16.855, 50.8966) -> (16.8327, 50.9423) centre (16.8439, 50.9195) ccw
  arc A898 (17.1121, 49.8351) -> (17.0664, 49.8129) centre (17.0892, 49.824) ccw
  arc A899 (1.1811, 32.1023) -> (1.2573, 32.1023) centre (1.2192, 32.1023) ccw
  line L227 (16.895, 50.2222) -> (16.7243, 50.5723)
  arc A900 (16.8327, 50.9423) -> (16.855, 50.8966) centre (16.8439, 50.9195) ccw
  arc A901 (17.0781, 49.8468) -> (17.1004, 49.8012) centre (17.0892, 49.824) ccw
  arc A902 (17.2849, 50.8457) -> (17.3305, 50.868) centre (17.3077, 50.8568) ccw
  arc A903 (17.1532, 49.783) -> (17.1989, 49.8052) centre (17.176, 49.7941) ccw
  line L228 (16.8438, 50.9195) -> (16.9605, 50.9764)
  line L229 (17.1761, 49.7941) -> (17.1476, 49.8525)
  arc A904 (16.7471, 50.5834) -> (16.7015, 50.5612) centre (16.7243, 50.5723) ccw
  arc A905 (2.3029, 32.5538) -> (2.032, 32.8248) centre (2.0319, 32.5538) ccw
  arc A906 (2.2648, 32.1023) -> (2.341, 32.1023) centre (2.3029, 32.1023) ccw
  arc A907 (17.6835, 51.329) -> (17.6378, 51.3067) centre (17.6606, 51.3178) ccw
  arc A908 (17.5005, 49.351) -> (17.4542, 49.0757) centre (17.6701, 49.1809) ccw
  arc A909 (24.5872, 10.9657) -> (24.5872, 11.0165) centre (24.5872, 10.9911) ccw
  line L230 (17.1177, 49.7657) -> (17.1761, 49.7941)
  line L231 (24.2909, 12.0626) -> (23.9945, 11.6675)
  arc A910 (23.6982, 11.6929) -> (23.6982, 11.6421) centre (23.6982, 11.6675) ccw
  line L232 (1.2192, 32.5538) -> (1.2192, 32.1023)
  arc A911 (24.5872, 11.6421) -> (24.5872, 11.6929) centre (24.5872, 11.6675) ccw
  arc A912 (1.1811, 32.5538) -> (1.2573, 32.5538) centre (1.2192, 32.5538) ccw
  arc A913 (1.4901, 32.8248) -> (1.2192, 32.5538) centre (1.4902, 32.5538) ccw
  arc A914 (2.032, 32.8629) -> (2.032, 32.7867) centre (2.032, 32.8248) ccw
  arc A915 (23.9742, 11.6827) -> (24.0149, 11.6522) centre (23.9946, 11.6675) ccw
  arc A916 (2.032, 32.7867) -> (2.032, 32.8629) centre (2.032, 32.8248) ccw
  arc A917 (17.9223, 50.7233) -> (17.968, 50.7456) centre (17.9451, 50.7345) ccw
  arc A918 (24.1061, 11.8179) -> (24.1299, 11.8628) centre (24.118, 11.8403) ccw
  line L233 (17.9452, 50.7344) -> (17.6606, 51.3178)
  arc A919 (2.2648, 32.5538) -> (2.341, 32.5538) centre (2.3029, 32.5538) ccw
  arc A920 (23.7101, 12.085) -> (23.6863, 12.0401) centre (23.6982, 12.0626) ccw
  arc A921 (17.4314, 49.0646) -> (17.4771, 49.0868) centre (17.4543, 49.0757) ccw
  arc A922 (16.8438, 50.9195) -> (16.7243, 50.5723) centre (16.9577, 50.6861) ccw
  line L234 (17.4784, 50.5068) -> (17.9452, 50.7344)
  arc A923 (17.837, 49.6235) -> (17.5005, 49.351) centre (18.2591, 48.7582) ccw
  arc A924 (17.1704, 49.8636) -> (17.1248, 49.8413) centre (17.1476, 49.8525) ccw
  arc A925 (24.3698, 10.7601) -> (24.4095, 10.7283) centre (24.3896, 10.7442) ccw
  arc A926 (17.4771, 49.0868) -> (17.4314, 49.0646) centre (17.4543, 49.0757) ccw
  arc A927 (23.6982, 11.0165) -> (23.6982, 10.9657) centre (23.6982, 10.9911) ccw
  line L235 (17.0893, 49.824) -> (17.1177, 49.7657)
  arc A928 (7.62, 35.7124) -> (7.62, 35.4076) centre (7.62, 35.56) ccw
  arc A929 (9.0424, 49.53) -> (8.7376, 49.53) centre (8.89, 49.53) ccw
  arc A930 (2.134, 30.7532) -> (2.2009, 30.7897) centre (2.1675, 30.7715) ccw
  arc A931 (12.8524, 49.53) -> (12.5476, 49.53) centre (12.7, 49.53) ccw
  line L236 (11.43, 24.13) -> (11.43, 35.56)
  line L237 (2.3029, 32.1023) -> (2.3029, 32.5538)
  line L238 (11.43, 35.56) -> (7.62, 35.56)
  line L239 (8.89, 49.53) -> (8.89, 44.45)
  arc A932 (8.89, 44.6024) -> (8.89, 44.2976) centre (8.89, 44.45) ccw
  line L240 (8.89, 44.45) -> (12.7, 44.45)
  arc A933 (12.7, 44.2976) -> (12.7, 44.6024) centre (12.7, 44.45) ccw
  arc A934 (12.5476, 44.45) -> (12.8524, 44.45) centre (12.7, 44.45) ccw
  arc A935 (11.5824, 20.32) -> (11.2776, 20.32) centre (11.43, 20.32) ccw
  line L241 (29.21, 17.78) -> (12.7, 17.78)
  line L242 (11.43, 20.32) -> (7.62, 20.32)
  arc A936 (8.7376, 44.45) -> (9.0424, 44.45) centre (8.89, 44.45) ccw
  arc A937 (7.4676, 11.43) -> (7.7724, 11.43) centre (7.62, 11.43) ccw
  line L243 (12.7, 49.53) -> (8.89, 49.53)
  arc A938 (11.43, 11.2776) -> (11.43, 11.5824) centre (11.43, 11.43) ccw
  line L244 (12.7, 38.1) -> (29.21, 38.1)
  line L245 (12.7, 17.78) -> (12.7, 38.1)
  line L246 (2.3029, 29.4642) -> (2.3029, 30.0061)
  arc A939 (7.62, 11.5824) -> (7.62, 11.2776) centre (7.62, 11.43) ccw
  arc A940 (1.2573, 31.0876) -> (1.1811, 31.0876) centre (1.2192, 31.0876) ccw
  arc A941 (2.341, 30.0061) -> (2.2648, 30.0061) centre (2.3029, 30.0061) ccw
  arc A942 (2.7398, 31.3814) -> (2.6789, 31.3357) centre (2.7094, 31.3585) ccw
  line L247 (7.62, 24.13) -> (11.43, 24.13)
  arc A943 (7.7724, 20.32) -> (7.4676, 20.32) centre (7.62, 20.32) ccw
  arc A944 (12.5984, 17.78) -> (12.8016, 17.78) centre (12.7, 17.78) ccw
  arc A945 (12.8016, 38.1) -> (12.5984, 38.1) centre (12.7, 38.1) ccw
  arc A946 (11.2776, 11.43) -> (11.5824, 11.43) centre (11.43, 11.43) ccw
  arc A947 (7.4676, 24.13) -> (7.7724, 24.13) centre (7.62, 24.13) ccw
  arc A948 (7.62, 20.4724) -> (7.62, 20.1676) centre (7.62, 20.32) ccw
  arc A949 (7.62, 24.2824) -> (7.62, 23.9776) centre (7.62, 24.13) ccw
  line L248 (7.62, 20.32) -> (7.62, 11.43)
  arc A950 (7.7724, 35.56) -> (7.4676, 35.56) centre (7.62, 35.56) ccw
  line L249 (12.7, 44.45) -> (12.7, 49.53)
  arc A951 (11.43, 20.1676) -> (11.43, 20.4724) centre (11.43, 20.32) ccw
  line L250 (29.21, 38.1) -> (29.21, 17.78)
  arc A952 (29.21, 17.6784) -> (29.21, 17.8816) centre (29.21, 17.78) ccw
  arc A953 (12.7, 49.3776) -> (12.7, 49.6824) centre (12.7, 49.53) ccw
  arc A954 (2.8829, 30.9521) -> (2.8067, 30.9521) centre (2.8448, 30.9521) ccw
  arc A955 (12.7, 17.8816) -> (12.7, 17.6784) centre (12.7, 17.78) ccw
  arc A956 (2.2003, 30.7908) -> (2.1346, 30.7522) centre (2.1674, 30.7715) ccw
  arc A957 (11.2776, 24.13) -> (11.5824, 24.13) centre (11.43, 24.13) ccw
  line L251 (7.62, 35.56) -> (7.62, 24.13)
  arc A958 (11.5824, 35.56) -> (11.2776, 35.56) centre (11.43, 35.56) ccw
  arc A959 (11.43, 23.9776) -> (11.43, 24.2824) centre (11.43, 24.13) ccw
  arc A960 (12.7, 38.2016) -> (12.7, 37.9984) centre (12.7, 38.1) ccw
  arc A961 (2.3029, 29.0641) -> (2.3029, 29.1403) centre (2.3029, 29.1022) ccw
  line L252 (1.8965, 31.2682) -> (2.1675, 30.7715)
  line L253 (7.62, 11.43) -> (11.43, 11.43)
  arc A962 (1.4181, 30.5187) -> (1.4718, 30.5728) centre (1.445, 30.5458) ccw
  arc A963 (11.43, 35.4076) -> (11.43, 35.7124) centre (11.43, 35.56) ccw
  arc A964 (1.93, 24.4608) -> (1.8631, 24.4243) centre (1.8966, 24.4425) ccw
  line L254 (1.2192, 25.2971) -> (2.3029, 25.2971)
  arc A965 (29.1084, 17.78) -> (29.3116, 17.78) centre (29.21, 17.78) ccw
  arc A966 (8.89, 49.6824) -> (8.89, 49.3776) centre (8.89, 49.53) ccw
  arc A967 (29.3116, 38.1) -> (29.1084, 38.1) centre (29.21, 38.1) ccw
  line L255 (0.6773, 32.1023) -> (2.3029, 32.1023)
  line L256 (2.032, 32.8248) -> (1.4901, 32.8248)
  arc A968 (1.5804, 31.4869) -> (1.5804, 31.4107) centre (1.5804, 31.4488) ccw
  arc A969 (29.21, 37.9984) -> (29.21, 38.2016) centre (29.21, 38.1) ccw
  line L257 (11.43, 11.43) -> (11.43, 20.32)
  arc A970 (1.2192, 25.3352) -> (1.2192, 25.259) centre (1.2192, 25.2971) ccw
  arc A971 (1.8895, 27.4017) -> (1.8133, 27.4017) centre (1.8514, 27.4017) ccw
  line L258 (1.2192, 27.8081) -> (2.032, 27.8081)
  arc A972 (2.2648, 25.2971) -> (2.341, 25.2971) centre (2.3029, 25.2971) ccw
  arc A973 (2.032, 26.4189) -> (2.032, 26.3427) centre (2.032, 26.3808) ccw
  arc A974 (2.2648, 26.1099) -> (2.341, 26.1099) centre (2.3029, 26.1099) ccw
  arc A975 (1.2192, 27.4017) -> (1.8514, 27.4017) centre (1.5353, 27.4017) ccw
  line L259 (1.8514, 27.8081) -> (1.8514, 27.4017)
  arc A976 (2.2648, 27.1759) -> (2.341, 27.1759) centre (2.3029, 27.1759) ccw
  arc A977 (2.3029, 28.5223) -> (2.3029, 28.5985) centre (2.3029, 28.5604) ccw
  arc A978 (2.032, 27.8462) -> (2.032, 27.77) centre (2.032, 27.8081) ccw
  arc A979 (2.1223, 29.1403) -> (2.1223, 29.0641) centre (2.1223, 29.1022) ccw
  line L260 (1.2192, 27.4017) -> (1.2192, 27.8081)
  arc A980 (0.6773, 32.1404) -> (0.6773, 32.0642) centre (0.6773, 32.1023) ccw
  line L261 (2.3029, 29.1022) -> (2.1223, 29.1022)
  arc A981 (1.2192, 28.5985) -> (1.2192, 28.5223) centre (1.2192, 28.5604) ccw
  arc A982 (1.1811, 27.4017) -> (1.2573, 27.4017) centre (1.2192, 27.4017) ccw
  line L262 (2.032, 26.3808) -> (1.2192, 26.3808)
  arc A983 (1.2573, 27.4017) -> (1.1811, 27.4017) centre (1.2192, 27.4017) ccw
  arc A984 (1.8895, 27.8081) -> (1.8133, 27.8081) centre (1.8514, 27.8081) ccw
  line L263 (1.2192, 28.5604) -> (2.3029, 28.5604)
  arc A985 (2.2648, 28.5604) -> (2.341, 28.5604) centre (2.3029, 28.5604) ccw
  line L264 (2.3029, 28.5604) -> (2.3029, 29.1022)
  arc A986 (2.2648, 27.5372) -> (2.341, 27.5372) centre (2.3029, 27.5372) ccw
  arc A987 (2.3029, 27.5372) -> (2.032, 27.8081) centre (2.032, 27.5372) ccw
  line L265 (2.3029, 25.2971) -> (2.3029, 26.1099)
  arc A988 (2.3029, 25.8009) -> (2.3029, 25.8771) centre (2.3029, 25.839) ccw
  arc A989 (1.8133, 27.4017) -> (1.8895, 27.4017) centre (1.8514, 27.4017) ccw
  arc A990 (2.032, 26.3427) -> (2.032, 26.4189) centre (2.032, 26.3808) ccw
  arc A991 (2.032, 27.77) -> (2.032, 27.8462) centre (2.032, 27.8081) ccw
  arc A992 (1.2192, 27.8462) -> (1.2192, 27.77) centre (1.2192, 27.8081) ccw
  line L266 (1.2192, 25.839) -> (2.3029, 25.839)
  arc A993 (2.3029, 25.259) -> (2.3029, 25.3352) centre (2.3029, 25.2971) ccw
  arc A994 (1.2192, 25.8771) -> (1.2192, 25.8009) centre (1.2192, 25.839) ccw
  arc A995 (1.2573, 27.8081) -> (1.1811, 27.8081) centre (1.2192, 27.8081) ccw
  arc A996 (2.3029, 26.1099) -> (2.032, 26.3808) centre (2.032, 26.1099) ccw
  arc A997 (1.2192, 26.4189) -> (1.2192, 26.3427) centre (1.2192, 26.3808) ccw
  arc A998 (2.341, 26.1099) -> (2.2648, 26.1099) centre (2.3029, 26.1099) ccw
  arc A999 (2.341, 27.5372) -> (2.2648, 27.5372) centre (2.3029, 27.5372) ccw
  line L267 (2.3029, 27.5372) -> (2.3029, 27.1759)
  arc A1000 (2.341, 29.1022) -> (2.2648, 29.1022) centre (2.3029, 29.1022) ccw
  arc A1001 (8.75, 51.7377) -> (7.75, 50.7377) centre (8.75, 50.7377) ccw
  line L268 (7.0166, 48.0756) -> (0, 42.188)
  line L269 (35, 0) -> (35, 42.1884)
  arc A1002 (27.25, 50.7377) -> (26.25, 51.7377) centre (26.25, 50.7377) ccw
  arc A1003 (27.25, 49.7377) -> (27.9783, 48.0802) centre (29.5001, 49.7376) ccw
  arc A1004 (7.0166, 48.0756) -> (7.75, 49.7377) centre (5.4999, 49.7377) ccw
  line L270 (0, 0) -> (0, 42.188)
  arc A1005 (29.499, 3.2386) -> (29.499, 4.2386) centre (29.499, 3.7386) ccw
  line L271 (35, 0) -> (0, 0)
  arc A1006 (5.499, 3.2377) -> (5.499, 4.2377) centre (5.499, 3.7377) ccw
  line L272 (8.75, 51.7377) -> (26.25, 51.7377)
  line L273 (27.9783, 48.0802) -> (35, 42.1884)
  line L274 (27.25, 49.7377) -> (27.25, 50.7377)
  arc A1007 (5.499, 4.2377) -> (5.499, 3.2377) centre (5.499, 3.7377) ccw
  arc A1008 (29.499, 4.2386) -> (29.499, 3.2386) centre (29.499, 3.7386) ccw
  line L275 (7.75, 49.7377) -> (7.75, 50.7377)
  arc A1009 (30.8896, 17.155) -> (29.9244, 17.155) centre (30.407, 17.155) ccw
  arc A1010 (29.9244, 42.555) -> (30.8896, 42.555) centre (30.407, 42.555) ccw
  arc A1011 (4.5194, 40.015) -> (5.4846, 40.015) centre (5.002, 40.015) ccw
  arc A1012 (29.9244, 27.315) -> (30.8896, 27.315) centre (30.407, 27.315) ccw
  arc A1013 (29.9244, 12.075) -> (30.8896, 12.075) centre (30.407, 12.075) ccw
  arc A1014 (5.4846, 40.015) -> (4.5194, 40.015) centre (5.002, 40.015) ccw
  arc A1015 (29.9244, 6.995) -> (30.8896, 6.995) centre (30.407, 6.995) ccw
  arc A1016 (29.9244, 37.475) -> (30.8896, 37.475) centre (30.407, 37.475) ccw
  arc A1017 (29.9244, 17.155) -> (30.8896, 17.155) centre (30.407, 17.155) ccw
  arc A1018 (30.8896, 19.695) -> (29.9244, 19.695) centre (30.407, 19.695) ccw
  arc A1019 (29.9244, 9.535) -> (30.8896, 9.535) centre (30.407, 9.535) ccw
  arc A1020 (30.8896, 12.075) -> (29.9244, 12.075) centre (30.407, 12.075) ccw
  arc A1021 (4.5194, 40.015) -> (5.4846, 40.015) centre (5.002, 40.015) ccw
  arc A1022 (29.9244, 19.695) -> (30.8896, 19.695) centre (30.407, 19.695) ccw
  arc A1023 (4.5194, 29.855) -> (5.4846, 29.855) centre (5.002, 29.855) ccw
  arc A1024 (30.8896, 12.075) -> (29.9244, 12.075) centre (30.407, 12.075) ccw
  arc A1025 (30.8896, 40.015) -> (29.9244, 40.015) centre (30.407, 40.015) ccw
  arc A1026 (30.8896, 9.535) -> (29.9244, 9.535) centre (30.407, 9.535) ccw
  arc A1027 (30.8896, 42.555) -> (29.9244, 42.555) centre (30.407, 42.555) ccw
  arc A1028 (4.5194, 29.855) -> (5.4846, 29.855) centre (5.002, 29.855) ccw
  arc A1029 (30.8896, 42.555) -> (29.9244, 42.555) centre (30.407, 42.555) ccw
  arc A1030 (30.8896, 6.995) -> (29.9244, 6.995) centre (30.407, 6.995) ccw
  arc A1031 (30.8896, 40.015) -> (29.9244, 40.015) centre (30.407, 40.015) ccw
  arc A1032 (29.9244, 14.615) -> (30.8896, 14.615) centre (30.407, 14.615) ccw
  arc A1033 (29.9244, 19.695) -> (30.8896, 19.695) centre (30.407, 19.695) ccw
  arc A1034 (5.4846, 40.015) -> (4.5194, 40.015) centre (5.002, 40.015) ccw
  arc A1035 (29.9244, 40.015) -> (30.8896, 40.015) centre (30.407, 40.015) ccw
  arc A1036 (29.9244, 9.535) -> (30.8896, 9.535) centre (30.407, 9.535) ccw
  arc A1037 (29.9244, 6.995) -> (30.8896, 6.995) centre (30.407, 6.995) ccw
  arc A1038 (30.8896, 17.155) -> (29.9244, 17.155) centre (30.407, 17.155) ccw
  arc A1039 (30.8896, 14.615) -> (29.9244, 14.615) centre (30.407, 14.615) ccw
  arc A1040 (4.5194, 37.475) -> (5.4846, 37.475) centre (5.002, 37.475) ccw
  arc A1041 (30.8896, 9.535) -> (29.9244, 9.535) centre (30.407, 9.535) ccw
  arc A1042 (30.8896, 27.315) -> (29.9244, 27.315) centre (30.407, 27.315) ccw
  arc A1043 (30.8896, 29.855) -> (29.9244, 29.855) centre (30.407, 29.855) ccw
  arc A1044 (29.9244, 12.075) -> (30.8896, 12.075) centre (30.407, 12.075) ccw
  arc A1045 (29.9244, 42.555) -> (30.8896, 42.555) centre (30.407, 42.555) ccw
  arc A1046 (29.9244, 17.155) -> (30.8896, 17.155) centre (30.407, 17.155) ccw
  arc A1047 (29.9244, 40.015) -> (30.8896, 40.015) centre (30.407, 40.015) ccw
  arc A1048 (30.8896, 22.235) -> (29.9244, 22.235) centre (30.407, 22.235) ccw
  arc A1049 (29.9244, 22.235) -> (30.8896, 22.235) centre (30.407, 22.235) ccw
  arc A1050 (30.8896, 6.995) -> (29.9244, 6.995) centre (30.407, 6.995) ccw
  arc A1051 (9.017, 31.115) -> (9.017, 30.353) centre (9.017, 30.734) ccw
  line L276 (10.541, 33.274) -> (9.017, 33.274)
  arc A1052 (9.017, 28.575) -> (9.017, 27.813) centre (9.017, 28.194) ccw
  arc A1053 (10.541, 25.273) -> (10.541, 26.035) centre (10.541, 25.654) ccw
  arc A1054 (10.541, 32.893) -> (10.541, 33.655) centre (10.541, 33.274) ccw
  arc A1055 (9.017, 26.035) -> (9.017, 25.273) centre (9.017, 25.654) ccw
  arc A1056 (9.017, 33.655) -> (9.017, 32.893) centre (9.017, 33.274) ccw
  line L277 (10.541, 28.194) -> (9.017, 28.194)
  arc A1057 (10.541, 27.813) -> (10.541, 28.575) centre (10.541, 28.194) ccw
  line L278 (10.541, 30.734) -> (9.017, 30.734)
  line L279 (10.541, 28.194) -> (9.017, 28.194)
  arc A1058 (9.017, 31.115) -> (9.017, 30.353) centre (9.017, 30.734) ccw
  arc A1059 (9.017, 28.575) -> (9.017, 27.813) centre (9.017, 28.194) ccw
  arc A1060 (10.541, 25.273) -> (10.541, 26.035) centre (10.541, 25.654) ccw
  arc A1061 (10.541, 32.893) -> (10.541, 33.655) centre (10.541, 33.274) ccw
  arc A1062 (9.017, 26.035) -> (9.017, 25.273) centre (9.017, 25.654) ccw
  line L280 (10.541, 25.654) -> (9.017, 25.654)
  line L281 (10.541, 25.654) -> (9.017, 25.654)
  arc A1063 (9.017, 33.655) -> (9.017, 32.893) centre (9.017, 33.274) ccw
  arc A1064 (10.541, 30.353) -> (10.541, 31.115) centre (10.541, 30.734) ccw
  arc A1065 (10.541, 27.813) -> (10.541, 28.575) centre (10.541, 28.194) ccw
  line L282 (10.541, 33.274) -> (9.017, 33.274)
  line L283 (10.541, 30.734) -> (9.017, 30.734)
  arc A1066 (10.541, 30.353) -> (10.541, 31.115) centre (10.541, 30.734) ccw
  line L284 (25, 40.7282) -> (25, 41.0598)
  line L285 (25.2342, 40.494) -> (25, 40.7282)
  line L286 (27.54, 40.7282) -> (27.54, 41.0598)
  line L287 (25, 41.0598) -> (25.2342, 41.294)
  line L288 (27.7742, 40.494) -> (27.54, 40.7282)
  line L289 (27.54, 40.7282) -> (27.54, 41.0598)
  line L290 (27.54, 40.7282) -> (27.54, 41.0598)
  line L291 (28.1058, 41.294) -> (28.3401, 41.0598)
  line L292 (27.7742, 41.294) -> (28.1058, 41.294)
  line L293 (27.54, 41.0598) -> (27.7742, 41.294)
  line L294 (25, 41.0598) -> (25.2342, 41.294)
  line L295 (28.3401, 40.7282) -> (28.1058, 40.494)